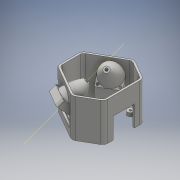
# Autodesk Inventor part: nozle mask front
Saved by Autodesk Inventor 2016 SP1 (Build 200210100, 210)
## iProperties
Created: 2016-04-21
Part Number: nozle mask front
Material: Generic
Document SubType Name: Modeling
Designer: ubik
Density: 1 g/cm^3
Appearance: Default
Author: ubik
Autodesk Inventor part; units mm, degrees
ref_plane "YZ Plane" through (0, 0, 0) normal (1, 0, 0) x (0, 1, 0)
ref_plane "XZ Plane" through (0, 0, 0) normal (0, 1, 0) x (-1, 0, 0)
ref_plane "XY Plane" through (0, 0, 0) normal (0, 0, 1) x (1, 0, 0)
sketch "Sketch1" plane through (0, 0, 0) normal (0, 0, 1) x (1, 0, 0)
  circle A0 centre (-21.75, -3) radius 1 projected
  circle A1 centre (-14.9186, 14) radius 1.5 projected
  circle A2 centre (-14.9186, -14) radius 1.5 projected
  circle A3 centre (21, 8.5) radius 1.5 projected
  circle A4 centre (9, 0) radius 1.5 projected
  circle A5 centre (21, -8.5) radius 1.5 projected
  circle A6 centre (12, -9) radius 6 projected
  circle A7 centre (12, 9) radius 6 projected
  circle A8 centre (5.9186, 35.7487) radius 2 projected
  circle A9 centre (-33.9186, 12.7487) radius 2 projected
  circle A10 centre (-33.9186, -12.7487) radius 2 projected
  circle A11 centre (5.9186, -35.7487) radius 2 projected
  circle A12 centre (28, -23) radius 2 projected
  circle A13 centre (28, 23) radius 2 projected
  line L0 (27, -14.75) -> (7, -14.75) projected
  line L1 (7, 14.75) -> (27, 14.75) projected
  circle A14 centre (28, -23) radius 5
  circle A15 centre (5.9186, -35.7487) radius 5
  circle A16 centre (28, 23) radius 5
  circle A17 centre (5.9186, 35.7487) radius 5
  line L2 (-41.9186, 0) -> (-41.9186, -12.7487)
  arc A18 (-41.9186, -12.7487) -> (-37.9186, -19.6769) centre (-33.9186, -12.7487) ccw
  line L3 (-37.9186, -19.6769) -> (1.9186, -42.6769)
  arc A19 (1.9186, -42.6769) -> (9.9186, -42.6769) centre (5.9186, -35.7487) ccw
  line L4 (9.9186, -42.6769) -> (32, -29.9282)
  arc A20 (32, -29.9282) -> (36, -23) centre (28, -23) ccw
  circle A21 centre (28, -23) radius 5.5
  circle A22 centre (5.9186, -35.7487) radius 5.5
  arc A23 (30.75, -27.7631) -> (33.5, -23) centre (28, -23) ccw
  line L5 (30.75, -27.7631) -> (8.6686, -40.5119)
  arc A24 (3.1686, -40.5119) -> (8.6686, -40.5119) centre (5.9186, -35.7487) ccw
  line L6 (3.1686, -40.5119) -> (-36.6686, -17.5119)
  arc A25 (-39.4186, -12.7487) -> (-36.6686, -17.5119) centre (-33.9186, -12.7487) ccw
  line L7 (-39.4186, -12.7487) -> (-39.4186, 0)
  line L8 (36, -15.25) -> (7, -15.25)
  line L9 (33.5, -15.25) -> (33.5, -23)
  line L10 (36, -23) -> (36, -15.25)
  line L11 (-57.1316, 0) -> (50.3748, 0) construction
  line L12 (-41.9186, 0) -> (-39.4186, 0)
  line L13 (36, -23) -> (36, 23) projected
  arc A26 (36, 23) -> (32, 29.9282) centre (28, 23) ccw projected
  line L14 (32, 29.9282) -> (9.9186, 42.6769) projected
  arc A27 (9.9186, 42.6769) -> (1.9186, 42.6769) centre (5.9186, 35.7487) ccw projected
  line L15 (1.9186, 42.6769) -> (-37.9186, 19.6769) projected
  arc A28 (-37.9186, 19.6769) -> (-41.9186, 12.7487) centre (-33.9186, 12.7487) ccw projected
  line L16 (-41.9186, 12.7487) -> (-41.9186, -12.7487) projected
  arc A29 (-41.9186, -12.7487) -> (-37.9186, -19.6769) centre (-33.9186, -12.7487) ccw projected
  line L17 (-37.9186, -19.6769) -> (1.9186, -42.6769) projected
  arc A30 (1.9186, -42.6769) -> (9.9186, -42.6769) centre (5.9186, -35.7487) ccw projected
  line L18 (9.9186, -42.6769) -> (32, -29.9282) projected
  arc A31 (32, -29.9282) -> (36, -23) centre (28, -23) ccw projected
  circle A32 centre (-33.4186, -0.7261) radius 1.5 projected
  circle A33 centre (16.0805, 29.3044) radius 1.5 projected
  circle A34 centre (17.3381, -28.5783) radius 1.5 projected
  circle A35 centre (-13.1686, 3) radius 1 projected
  point P0 (0, 0)
  point P1 (-12.8721, -34.1375)
  point P2 (-12.8721, -31.2507)
  dimension "d3" = 0.5
  dimension "d4" = 0.5
  dimension "d7" = 0.5
  constraints: 22 end point, 12 centre point, 12 point on circle, 5 point on line, 1 horizontal, 1 parallel, 4 other
  measures "d3" radial gap between concentric circles of A14 A21
  measures "d4" radial gap between concentric circles of A15 A22
  measures "d7" distance between parallel lines of L0 L8
extrude "Extrusion1" add sketch "Sketch1" along normal blind 10 contours L12 L7 A25 L6 A22 L5 A21 L9 L8 L10 A20 L4 A19 L3 A18 L2
ref_plane "Work Plane1" through (-15.7131, -36.1715, 28.0312) normal (0.3535534, 0.6123724, 0.7071068) x (0.8660254, -0.5, 0)
sketch "Sketch3" plane through (-15.7131, -36.1715, 28.0312) normal (0.3535534, 0.6123724, 0.7071068) x (0.8660254, -0.5, 0)
  line L0 (-12.5, 15) -> (12.5, 15) projected
  arc A0 (-12.5, 15) -> (-15, 12.5) centre (-12.5, 12.5) ccw projected
  line L1 (-15, 12.5) -> (-15, -12.5) projected
  arc A1 (-15, -12.5) -> (-12.5, -15) centre (-12.5, -12.5) ccw projected
  line L2 (-12.5, -15) -> (12.5, -15) projected
  arc A2 (12.5, -15) -> (15, -12.5) centre (12.5, -12.5) ccw projected
  line L3 (15, 12.5) -> (15, -12.5) projected
  arc A3 (15, 12.5) -> (12.5, 15) centre (12.5, 12.5) ccw projected
  circle A4 centre (0, 0) radius 14.375 projected
  circle A5 centre (-12, -12) radius 1.75 projected
  circle A6 centre (-12, 12) radius 1.75 projected
  circle A7 centre (12, -12) radius 1.75 projected
  circle A8 centre (12, 12) radius 1.75 projected
  line L4 (0, 22.779) -> (0, -22.2099)
  point P0 (-4.4778, 47.5269)
  constraints: 2 end point, 1 vertical
ref_plane "Work Plane2" through (-15.7131, -36.1715, 28.0312) normal (0.8660254, -0.5, 0) x (0.3535534, 0.6123724, 0.7071068)
ref_plane "Work Plane3" through (10.25, -12.0311, 55) normal (0, 0, 1) x (1, 0, 0)
sketch "Sketch5" plane through (-15.7131, -36.1715, 28.0312) normal (0.8660254, -0.5, 0) x (0.3535534, 0.6123724, 0.7071068)
  line L0 (0.0278, -14.3239) -> (0.0278, -13.5559)
  line L1 (-72.0235, 0) -> (108.8939, 0) projected
  arc A0 (0.0278, -14.3239) -> (35.9865, -1.9308) centre (-0.1447, 44.5401) ccw
  arc A1 (0.0278, -15.8239) -> (35.9865, -3.8168) centre (-0.1447, 44.5401) ccw
  line L2 (35.9865, -1.9308) -> (35.9865, -3.8168)
  line L3 (0.0278, -14.3239) -> (0.0278, -15.8239)
  point P0 (7.8848, -47.5269)
  dimension "d13" = 1.5
  constraints: 6 end point, 4 point on circle, 2 centre point, 2 vertical, 1 parallel
  measures "d13" radial gap between concentric circles of A0 A1
revolve "Revolution2" add sketch "Sketch5" angle 360 about axis through (-15.7131, -36.1715, 28.0312) along (0.3535534, 0.6123724, 0.7071068)
extrude "Extrusion4" add sketch "Sketch3" along normal blind 10 contours L0 L4 A4 L2 A1 L1 A0 | L0 A3 L3 A2 L2 L4 A4
sketch "Sketch7" plane through (0, 0, 0) normal (0, 0, -1) x (-1, 0, 0)
  ellipse E0 centre (15.7131, -36.1715) end of major axis (28.1622, -28.984) minor radius 10.1647 (23.1946, -25.2911) -> (2.5497, -37.2104) ccw
  line L0 (-1.6967, -36.0168) -> (-0.1183, -38.7507)
  line L1 (10.1911, -51.6071) -> (31.8417, -39.1071) projected
  line L2 (25.8625, -23.7507) -> (24.2841, -21.0168)
  line L3 (-3.1686, -40.5119) -> (25.8625, -23.7507)
  line L4 (-3.951, -27.1122) -> (17.6996, -14.6122)
  ellipse E1 centre (18.5835, -16.1431) end of major axis (16.4184, -17.3931) minor radius 1.7678 (20.7485, -14.8931) -> (17.6996, -14.6122) ccw
  ellipse E2 centre (-3.0672, -28.6431) end of major axis (-0.9021, -27.3931) minor radius 1.7678 (-3.951, -27.1122) -> (-5.2322, -29.8931) ccw
  line L5 (24.2841, -21.0168) -> (20.7485, -14.8931) projected
  line L6 (24.2841, -21.0168) -> (20.7485, -14.8931)
  line L7 (20.7485, -14.8931) -> (29.5874, -30.2024) projected
  ellipse E3 centre (-3.0672, -28.6431) end of major axis (-0.9021, -27.3931) minor radius 1.7678 (-3.951, -27.1122) -> (-5.2322, -29.8931) ccw projected
  line L8 (-1.6967, -36.0168) -> (-5.2322, -29.8931)
  point P0 (0, 0)
  constraints: 12 end point, 3 point on line, 1 collinear, 13 other
extrude "Extrusion5" add sketch "Sketch7" against normal up to surface surface through (0.4155, -33.2359, 17.4246) normal (0.3535534, 0.6123724, -0.7071068)
sketch "Sketch8" plane through (-15.7131, -36.1715, 28.0312) normal (-0.3535534, -0.6123724, -0.7071068) x (-0.8660254, 0.5, 0)
  line L0 (15, 5.0396) -> (15, -5.0396) projected
  arc A0 (15, -5.0396) -> (15, 5.0396) centre (0, 0) ccw projected
  arc A1 (-15, 5.0396) -> (-15, -5.0396) centre (0, 0) ccw projected
  line L1 (-15, 12.5) -> (-15, -12.5) projected
  circle A2 centre (-12, -12) radius 1.75 projected
  arc A3 (-12.0548, -10.2509) -> (-10.2509, -12.0548) centre (0, 0) ccw projected
  arc A4 (-5.0396, -15) -> (5.0396, -15) centre (0, 0) ccw projected
  line L2 (-12.5, -15) -> (12.5, -15) projected
  circle A5 centre (12, -12) radius 1.75 projected
  arc A6 (10.2509, -12.0548) -> (12.0548, -10.2509) centre (0, 0) ccw projected
  circle A7 centre (12, 12) radius 1.75 projected
  arc A8 (12.0548, 10.2509) -> (10.2509, 12.0548) centre (0, 0) ccw projected
  arc A9 (-10.2509, 12.0548) -> (-12.0548, 10.2509) centre (0, 0) ccw projected
  circle A10 centre (-12, 12) radius 1.75 projected
  point P0 (4.4778, 47.5269)
extrude "Extrusion6" cut sketch "Sketch8" against normal blind 10 contours A0 L0 | L1 A1 | A2 A3 | L2 A4 | A6 A5 | A8 A7 | A10 A9 picked at (-11.0057, -11.087) picked at (11.0952, -10.9991) picked at (11.0952, 10.9991) picked at (-11.0057, 11.087)
sketch "Sketch9" plane through (-15.7131, -36.1715, 28.0312) normal (-0.3535534, -0.6123724, -0.7071068) x (-0.8660254, 0.5, 0)
  arc A0 (15, 12.5) -> (12.5, 15) centre (12.5, 12.5) ccw
  arc A1 (-12.5, 15) -> (-15, 12.5) centre (-12.5, 12.5) ccw
  line L0 (-15, 15) -> (-15, 12.5)
  line L1 (15, 12.5) -> (15, 15)
  line L2 (12.5, 15) -> (-12.5, 15) projected
  line L3 (-12.5, 15) -> (-15, 15)
  line L4 (12.5, 15) -> (15, 15)
  point P0 (4.4778, 47.5269)
  point P1 (-1.4434, 15)
  constraints: 8 end point, 6 point on circle, 2 centre point, 1 collinear
extrude "Extrusion7" add sketch "Sketch9" against normal blind 10
sketch "Sketch10" plane through (0, 0, 0) normal (0, 0, -1) x (-1, 0, 0)
  ellipse E0 centre (18.5835, -16.1431) end of major axis (20.7485, -14.8931) minor radius 1.7678 (20.7485, -14.8931) -> (17.6996, -14.6122) ccw projected
  line L0 (20.7485, -14.8931) -> (19.8647, -13.3622) projected
  line L1 (17.6996, -14.6122) -> (19.8647, -13.3622) projected
  ellipse E1 centre (-3.0672, -28.6431) end of major axis (-5.2322, -29.8931) minor radius 1.7678 (-3.951, -27.1122) -> (-5.2322, -29.8931) ccw projected
  line L2 (-6.1161, -28.3622) -> (-3.951, -27.1122) projected
  line L3 (-5.2322, -29.8931) -> (-6.1161, -28.3622) projected
  point P0 (0, 0)
  constraints: 2 other
extrude "Extrusion8" add sketch "Sketch10" against normal up to next
sketch "Sketch11" plane through (0, 0, 10) normal (0, 0, 1) x (1, 0, 0)
  line L0 (-1.1317, -40.9158) -> (1.9186, -42.6769)
  arc A0 (1.9186, -42.6769) -> (9.9186, -42.6769) centre (5.9186, -35.7487) ccw
  line L1 (9.9186, -42.6769) -> (32, -29.9282) projected
  arc A1 (32, -29.9282) -> (36, -23) centre (28, -23) ccw projected
  line L2 (36, -23) -> (36, -15.25) projected
  line L3 (36, -15.25) -> (33.5, -15.25) projected
  line L4 (33.5, -15.25) -> (33.5, -23) projected
  line L5 (30.75, -27.7631) -> (8.6686, -40.5119) projected
  line L6 (3.1686, -40.5119) -> (0.1183, -38.7507)
  line L7 (-1.1317, -40.9158) -> (0.1183, -38.7507)
  arc A2 (3.1686, -40.5119) -> (8.6686, -40.5119) centre (5.9186, -35.7487) ccw projected
  arc A3 (30.75, -27.7631) -> (33.5, -23) centre (28, -23) ccw projected
  point P0 (0, 0)
  constraints: 6 end point, 3 centre point, 2 point on circle
extrude "Extrusion10" add sketch "Sketch11" along normal blind 45
sketch "Sketch12" plane through (0.1183, -38.7507, 36.4914) normal (-0.8660254, 0.5, 0) x (0, 0, 1)
  line L0 (-36.4914, 2.75) -> (-36.4914, 0) projected
  line L1 (-36.4914, 0) -> (18.5086, 0)
  line L2 (-36.4914, 2.75) -> (-2.75, 2.75)
  line L3 (2.5, -2.5) -> (0, 0)
  line L4 (2.5, -2.5) -> (18.5086, -2.5)
  line L5 (18.5086, 0) -> (18.5086, -2.5)
  line L6 (0, 0) -> (18.5086, 0) projected
  point P0 (-36.4914, 33.5)
  constraints: 10 end point
extrude "Extrusion11" add sketch "Sketch12" along normal blind 45
sketch "Sketch14" plane through (-24.7455, -27.2824, 38.9914) normal (-0.5, -0.8660254, 0) x (0.8660254, -0.5, 0)
  spline S0 degree 5 poles (0, 0) (0.678, 1.498) (1.5085, 2.9258) (2.4981, 4.2583) (3.6454, 5.4562) (6.192, 7.4416) (7.5784, 8.2409) (9.0896, 8.8177) (10.6751, 9.106) (13.8519, 9.1081) (15.4453, 8.8191) (16.9637, 8.2387) (18.3558, 7.4339) (20.3109, 5.9046) (20.9678, 5.3021) (21.5796, 4.6532) (22.1453, 3.9651) (22.8896, 2.9328) (23.1054, 2.6156) (23.3126, 2.2927) (23.5114, 1.9645) (23.7929, 1.4719) (23.8821, 1.3113) (23.9694, 1.1496) (24.0547, 0.9868) (24.2217, 0.659) (24.3029, 0.495) (24.3818, 0.3308) (24.4586, 0.1659) (24.5337, 0) knots 0 0 0 0 0 0 0.254262 0.254262 0.254262 0.254262 0.499692 0.499692 0.499692 0.499692 0.746291 0.746291 0.746291 0.746291 0.883799 0.883799 0.883799 0.883799 0.943111 0.943111 0.943111 0.943111 0.971521 0.971521 0.971521 0.971521 1 1 1 1 1 1 projected
  line L0 (24.5337, 0) -> (0, 0) projected
  point P0 (7.7891, -38.9914)
  constraints: 1 horizontal alignment
extrude "Extrusion12" cut sketch "Sketch14" against normal up to surface (2.5 mm away)
sketch "Sketch16" plane through (0, 0, 10) normal (0, 0, 1) x (1, 0, 0)
  line L0 (-1.1317, -40.9158) -> (0.1183, -38.7507) projected
  line L1 (0.1183, -38.7507) -> (-25.8625, -23.7507) projected
  line L2 (-25.8625, -23.7507) -> (-36.6686, -17.5119) projected
  arc A0 (-39.4186, -12.7487) -> (-36.6686, -17.5119) centre (-33.9186, -12.7487) ccw projected
  line L3 (-39.4186, -12.7487) -> (-39.4186, 0) projected
  line L4 (-39.4186, 0) -> (-41.9186, 0) projected
  line L5 (-41.9186, 0) -> (-41.9186, -12.7487) projected
  arc A1 (-41.9186, -12.7487) -> (-37.9186, -19.6769) centre (-33.9186, -12.7487) ccw projected
  line L6 (-37.9186, -19.6769) -> (-1.1317, -40.9158) projected
  line L7 (-25.8625, -23.7507) -> (-27.1125, -25.9158) projected
  point P0 (0, 0)
extrude "Extrusion14" add sketch "Sketch16" along normal up to surface (45 mm away) contours L6 A1 L5 L4 L3 A0 L2 L7
sketch "Sketch17" plane through (33.5, -15.25, 0) normal (0, 1, 0) x (1, 0, 0)
  line L0 (0, 0) -> (2.5, 0) projected
  line L1 (0, -30) -> (0, -55)
  line L2 (2.5, -55) -> (0, -55) projected
  line L3 (2.5, -30) -> (2.5, -55)
  line L4 (0, -30) -> (2.5, -30)
  point P0 (-33.5, 0)
  dimension "d41" = 25
  constraints: 6 end point, 1 perpendicular
  measures "d41" distance between parallel lines of L4 L2
extrude "Extrusion15" add sketch "Sketch17" along normal blind 16
mirror "Mirror2" about plane through (0, 0, 0) normal (0, 1, 0) of "Extrusion1", "Revolution2", "Extrusion4", "Extrusion5", "Extrusion6", "Extrusion7", "Extrusion8", "Extrusion10", "Extrusion11", "Extrusion12", "Extrusion14", "Extrusion15"
sketch "Sketch18" plane through (0, 0, 0) normal (0, 0, -1) x (-1, 0, 0)
  circle A0 centre (-5.9186, 35.7487) radius 5 projected
  circle A1 centre (-5.9186, -35.7487) radius 5.5 projected
  point P0 (0, 0)
extrude "Extrusion16" cut sketch "Sketch18" against normal blind 10
sketch "Sketch19" plane through (0, 0, 0) normal (0, 0, -1) x (-1, 0, 0)
  arc A0 (-19.9776, 27.0544) -> (-12.1834, 31.5544) centre (-16.0805, 29.3044) ccw
  line L0 (-22.9776, 32.2505) -> (-15.1834, 36.7505)
  line L1 (-19.9776, 27.0544) -> (-22.9776, 32.2505)
  line L2 (-12.1834, 31.5544) -> (-15.1834, 36.7505)
  circle A1 centre (-16.0805, 29.3044) radius 1.5
  line L3 (-21.2352, -26.3283) -> (-24.2352, -31.5245)
  line L4 (-16.441, -36.0245) -> (-24.2352, -31.5245)
  line L5 (-13.441, -30.8283) -> (-16.441, -36.0245)
  arc A2 (-13.441, -30.8283) -> (-21.2352, -26.3283) centre (-17.3381, -28.5783) ccw
  circle A3 centre (-17.3381, -28.5783) radius 1.5
  line L6 (33.4186, -5.2261) -> (39.4186, -5.2261)
  line L7 (39.4186, 3.7739) -> (39.4186, -5.2261)
  line L8 (33.4186, 3.7739) -> (39.4186, 3.7739)
  arc A4 (33.4186, 3.7739) -> (33.4186, -5.2261) centre (33.4186, -0.7261) ccw
  circle A5 centre (33.4186, -0.7261) radius 1.5
  point P0 (0, 0)
  dimension "d46" = 9
  dimension "d47" = 6
  dimension "d48" = 3
  dimension "d51" = 360
  constraints: 18 end point, 6 centre point, 6 point on circle, 3 coincident, 2 perpendicular, 2 tangent, 34 other
  measures "d46" diameter of A0
  measures "d47" distance from line of L0 A0.centre
  measures "d48" diameter of A1
extrude "Extrusion17" add sketch "Sketch19" against normal blind 5
fillet "Fillet1" radius 2 6 edges at (22.9776, 32.2505, 2.5) (15.1834, 36.7505, 2.5) (-39.4186, 3.7739, 2.5) (-39.4186, -5.2261, 2.5) (24.2352, -31.5245, 2.5) (16.441, -36.0245, 2.5)
body "Solid1"
